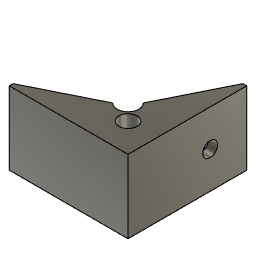
fan_mount (Autodesk Fusion 360 design; units mm, degrees)
Autodesk Fusion 360 part; units mm, degrees
sketch "Sketch1" plane through (0, 0, 0) normal (0, 0, 1) x (1, 0, 0)
  line L0 (0, 0) -> (-118.5, 0) construction
  line L1 (-118.5, 0) -> (-118.5, 118.5) construction
  line L2 (-118.5, 118.5) -> (0, 118.5) construction
  line L3 (0, 118.5) -> (0, 0) construction
  line L4 (0, 0) -> (-26, 0)
  line L5 (-26, 0) -> (-26, 26)
  line L6 (-26, 26) -> (0, 26)
  line L7 (0, 26) -> (0, 0)
  dimension "d11" = 118.5
  dimension "d12" = 118.5
  dimension "d13" = 26
  dimension "d14" = 26
  constraint horizontal L0
  constraint vertical L1
  constraint horizontal L2
  constraint vertical L3
  constraint coincident L0.start L3.end
  constraint horizontal L4
  constraint vertical L5
  constraint horizontal L6
  constraint vertical L7
  measures "d11" distance of L0.start L0.end
  measures "d12" distance of L0.start L2.end
  measures "d13" distance of L0.start L4.end
  measures "d14" distance of L0.start L6.end
extrude "Extrude1" add sketch "Sketch1" along normal blind 16
sketch "Sketch2" plane through (0, 0, 16) normal (0, 0, 1) x (-1, 0, 0)
  line L0 (0, -26) -> (26, -26)
  line L1 (26, -26) -> (26, 0)
  line L2 (26, 0) -> (0, 0)
  line L3 (0, 0) -> (0, -26)
  circle A0 centre (6.3, -6.3) radius 2
  dimension "d17" = 4
  dimension "d18" = 6.3
  dimension "d19" = 6.3
  measures "d17" diameter of A0
  measures "d18" distance of L3 A0.centre
  measures "d19" distance of L2 A0.centre
extrude "Extrude2" cut sketch "Sketch2" against normal up to surface (16 mm away) contours A0
sketch "Sketch3" plane through (0, 0, 0) normal (0, 0, 1) x (1, 0, 0)
  line L0 (0, 0) -> (-118.5, 0) construction
  line L1 (-118.5, 0) -> (-118.5, 118.5) construction
  line L2 (-118.5, 118.5) -> (0, 118.5) construction
  line L3 (0, 118.5) -> (0, 0) construction
  line L4 (-118.5, 59.25) -> (0, 59.25) construction
  line L5 (-59.25, 118.5) -> (-59.25, 0) construction
  circle A0 centre (-59.25, 59.25) radius 66.5
  dimension "d22" = 118.5
  dimension "d23" = 118.5
  dimension "d24" = 133
  constraint horizontal L0
  constraint vertical L1
  constraint horizontal L2
  constraint vertical L3
  constraint coincident L0.start L3.end
  constraint midpoint L1 L4.start
  constraint midpoint L3 L4.end
  constraint midpoint L2 L5.start
  constraint midpoint L0 L5.end
  constraint midpoint L4 A0.centre
  measures "d22" distance of L0.start L2.end
  measures "d23" distance of L0.start L0.end
  measures "d24" diameter of A0
extrude "Extrude3" cut sketch "Sketch3" along normal up to surface (16 mm away)
sketch "Sketch4" plane through (0, 0, 0) normal (0, 0, 1) x (1, 0, 0)
  line L0 (-8.0678, 11.4265) -> (-18.8511, 22.2099)
  arc A0 (-18.8511, 22.2099) -> (-22.2099, 18.8511) centre (-20.5305, 20.5305) ccw
  line L1 (-22.2099, 18.8511) -> (-11.4265, 8.0678)
  arc A1 (-11.4265, 8.0678) -> (-8.0678, 11.4265) centre (-9.7471, 9.7471) ccw
  line L2 (-8.0678, 8.0678) -> (-22.2099, 22.2099) construction
  circle A2 centre (-6.3, 6.3) radius 2
  dimension "d27" = 4.75
  dimension "d28" = 2.5
  constraint tangent L0 A0
  constraint tangent A0 L1
  constraint parallel L0 L1
  constraint tangent L1 A1
  constraint tangent L0 A1
  constraint midpoint A1 L2.start
  constraint midpoint A0 L2.end
  measures "d27" diameter of A0
  measures "d28" distance of L2.start A2.centre
extrude "Extrude4" cut sketch "Sketch4" along normal up to surface (16 mm away) contours L0 A0 L1 A1
sketch "Sketch5" plane through (0, 0, 0) normal (0, 0, 1) x (1, 0, 0)
sketch "Sketch6" plane through (0, 0, 16) normal (0, 0, 1) x (-1, 0, 0)
  circle A0 centre (6.3, -6.3) radius 2
  line L0 (10.578, -13.9368) -> (8.0678, -11.4265)
  arc A1 (11.4265, -8.0678) -> (8.0678, -11.4265) centre (9.7471, -9.7471) ccw
  line L1 (11.4265, -8.0678) -> (13.9368, -10.578)
  arc A2 (26, -1.6593) -> (13.9368, -10.578) centre (59.25, -59.25) ccw
  line L2 (26, -1.6593) -> (26, 0)
  line L3 (26, 0) -> (0, 0)
  line L4 (0, 0) -> (0, -26)
  line L5 (0, -26) -> (1.6593, -26)
  arc A3 (10.578, -13.9368) -> (1.6593, -26) centre (59.25, -59.25) ccw
  line L6 (11.4265, -8.0678) -> (26, -0.8297)
  line L7 (26, -1.6593) -> (13.9368, -10.578)
  line L8 (13.9368, -10.578) -> (11.4265, -8.0678)
  line L9 (26, -1.6593) -> (26, -0.8297)
  constraint coincident A1.start L1.start
  constraint midpoint L2 L6.end
  constraint coincident A2.start L2.start
  constraint coincident L1.end A2.end
extrude "Extrude5" cut sketch "Sketch6" against normal up to surface (16 mm away) contours L1 A2 L2 L6 L8 L9
sketch "Sketch7" plane through (0, 0, 16) normal (0, 0, 1) x (-1, 0, 0)
  line L0 (11.4265, -8.0678) -> (26, -0.8297)
  line L1 (26, -0.8297) -> (26, 0)
  line L2 (26, 0) -> (0, 0)
  line L3 (0, 0) -> (0, -26)
  line L4 (0, -26) -> (1.6593, -26)
  arc A0 (10.578, -13.9368) -> (1.6593, -26) centre (59.25, -59.25) ccw
  line L5 (10.578, -13.9368) -> (8.0678, -11.4265)
  arc A1 (11.4265, -8.0678) -> (8.0678, -11.4265) centre (9.7471, -9.7471) ccw
  circle A2 centre (6.3, -6.3) radius 2
  line L6 (8.0678, -11.4265) -> (0.8297, -26)
  line L7 (0.8297, -26) -> (1.6593, -26)
  line L8 (1.6593, -26) -> (10.578, -13.9368)
  line L9 (10.578, -13.9368) -> (8.0678, -11.4265)
  constraint coincident L5.end A1.end
  constraint midpoint L4 L6.end
  constraint coincident L4.end A0.end
  constraint coincident A0.start L5.start
extrude "Extrude6" cut sketch "Sketch7" against normal up to surface (16 mm away) contours L4 A0 L5 L6 L7 L9
sketch "Sketch8" plane through (0, 0, 0) normal (1, 0, 0) x (0, 1, 0)
  line L0 (0, 0) -> (26, 0)
  line L1 (26, 0) -> (26, 16)
  line L2 (26, 16) -> (0, 16)
  line L3 (0, 16) -> (0, 0)
  circle A0 centre (18, 8) radius 1.625
  dimension "d39" = 3.25
  dimension "d40" = 18
  measures "d39" diameter of A0
  measures "d40" distance of L3 A0.centre
extrude "Extrude7" cut sketch "Sketch8" along normal up to surface contours A0 end surface through (-8.0678, 11.4265, 16) normal (-0.895619, 0.444821, 0) offset 0
sketch "Sketch9" plane through (0, 0, 0) normal (1, 0, 0) x (0, 1, 0)
  circle A0 centre (18, 8) radius 1.625
  line L0 (0, 0) -> (26, 0)
  line L1 (26, 0) -> (26, 16)
  line L2 (26, 16) -> (0, 16)
  line L3 (0, 16) -> (0, 0)
  line L4 (21.25, 5.2) -> (14.75, 5.2)
  line L5 (14.75, 5.2) -> (14.75, 10.8)
  line L6 (14.75, 10.8) -> (21.25, 10.8)
  line L7 (21.25, 10.8) -> (21.25, 5.2)
  line L8 (21.25, 5.2) -> (14.75, 10.8) construction
  line L9 (14.75, 5.2) -> (21.25, 10.8) construction
  point P0 (18, 8)
  dimension "d46" = 6.5
  dimension "d47" = 5.6
  constraint perpendicular L4 L5
  constraint parallel L4 L6
  constraint parallel L5 L7
  constraint horizontal L4
  constraint coincident L8 P0
  constraint coincident L9 P0
  constraint coincident P0 A0.centre
  measures "d46" distance of L5.end L6.end
  measures "d47" distance of L4.end L5.end
extrude "Extrude8" cut sketch "Sketch9" along normal up to surface from surface at -2 contours L4 L5 L6 L7 end surface through (-8.0678, 11.4265, 16) normal (-0.895619, 0.444821, 0) offset 0
equation "fan_mount_hole_diameter = 4 mm"
equation "fan_mount_length = 26 mm"
equation "fan_mount_width = 16 mm"
equation "fan_mount_height = 26 mm"
equation "fan_inner_diameter = 115.2 mm"
equation "fan_mount_hole_edge_offset = 4.3 mm + ( fan_mount_hole_diameter / 2 )"
equation "fan_outer_mount_strut_width = 4.75 mm"
equation "fan_cove_radius = 66.5 mm"
equation "fan_mount_hole_cove_offset = 6 mm"
equation "fan_overall_width = 118.5 mm"
equation "d11 = fan_overall_width"
equation "d12 = fan_overall_width"
equation "d13 = fan_mount_length"
equation "d14 = fan_mount_height"
equation "d15 = fan_mount_width"
equation "d17 = fan_mount_hole_diameter"
equation "d18 = fan_mount_hole_edge_offset"
equation "d19 = fan_mount_hole_edge_offset"
equation "d22 = fan_overall_width"
equation "d23 = fan_overall_width"
equation "d24 = 2 * fan_cove_radius"
equation "d27 = fan_outer_mount_strut_width"
equation "d28 = ( fan_mount_hole_diameter / 2 ) + fan_strut_hole_offset"
equation "fan_strut_hole_offset = 0.5 mm"
equation "sharp_corner_fillet = 2 mm"
equation "bottom_hole_diameter = 3.25 mm"
equation "bottom_hole_edge_offset = 18 mm"
equation "d39 = bottom_hole_diameter"
equation "d40 = bottom_hole_edge_offset"
equation "bottom_screw_mount_nut_holder_width = 5.6 mm"
equation "bottom_screw_mount_nut_holder_length = 6.5 mm"
equation "bottom_screw_mount_nut_holder_bottom_offset = 2 mm"
equation "d46 = bottom_screw_mount_nut_holder_length"
equation "d47 = bottom_screw_mount_nut_holder_width"
equation "d48 = -bottom_screw_mount_nut_holder_bottom_offset"
